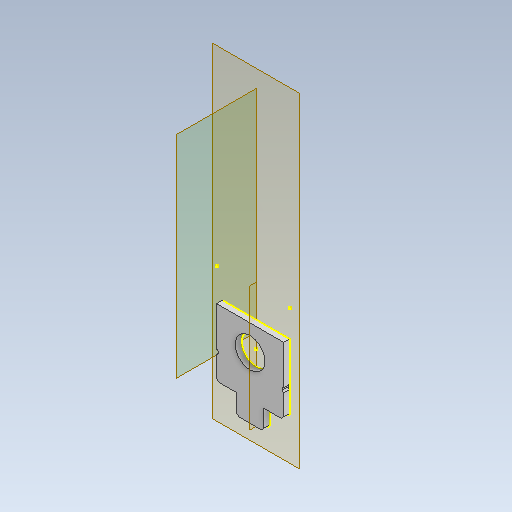
# Autodesk Inventor part: internal
Saved by Autodesk Inventor 2020 (Build 240168000, 168)
## iProperties
Created: 2020-02-17
Part Number: internal
Material: Generic
Document SubType Name: Modeling
Designer: erwin
Density: 1 g/cm^3
Appearance: Default
Mass: 213.639 g
Surface Area: 453.068 cm^2
Volume: 213.639 cm^3
Author: erwin
Autodesk Inventor part; units mm, degrees
ref_plane "YZ Plane" through (0, 0, 0) normal (1, 0, 0) x (0, 1, 0)
ref_plane "XZ Plane" through (0, 0, 0) normal (0, 1, 0) x (-1, 0, 0)
ref_plane "XY Plane" through (0, 0, 0) normal (0, 0, 1) x (1, 0, 0)
ref_plane "Work Plane1" through (0, 0, 0) normal (0, 0, 1) x (1, 0, 0)
sketch "Sketch1" plane through (0, 0, 0) normal (0, 0, 1) x (1, 0, 0)
  circle A0 centre (-67.9848, -106.1458) radius 30 projected
  line L0 (0, -139.7083) -> (0, -24) projected
  line L1 (-95.6323, -230.1458) -> (-40.3675, -230.1458)
  line L2 (-40.3675, -230.1458) -> (-40.3675, -106.1458)
  line L3 (-40.3675, -106.1458) -> (-95.6323, -106.1458)
  line L4 (-95.6323, -106.1458) -> (-95.6323, -230.1458)
  line L5 (-135.9998, -189.7783) -> (0, -189.7783)
  line L6 (0, -189.7783) -> (0, -53.7785)
  line L7 (0, -53.7785) -> (-135.9998, -53.7785)
  line L8 (-135.9998, -53.7785) -> (-135.9998, -189.7783)
  line L9 (-147.9998, -163.7083) -> (-135.9998, -163.7083) projected
  line L10 (-135.9998, -189.7783) -> (-135.9998, -163.7083) projected
  line L11 (-135.9998, -189.7783) -> (-147.9998, -189.7783) projected
  line L12 (-147.9998, -189.7783) -> (-147.9998, -163.7083) projected
  point P0 (0, 0)
  point P1 (-40.3675, -230.1458)
  point P2 (0, -189.7783)
  point P3 (-40.3675, -189.7783)
  point P4 (-95.6323, -189.7783)
  constraints: 16 end point, 4 parallel, 3 perpendicular, 2 collinear, 2 horizontal, 1 point on line, 3 other
extrude "Extrusion1" add sketch "Sketch1" along normal blind 12 contours A0 L4 L5 L8 L7 L0 L6 L2 | A0 L2 L5 L4 | L5 L2 L1 L4
chamfer "Chamfer1" distance 5 angle 45 4 edges at (-135.9998, -189.7783, 6) (-95.6323, -230.1458, 6) (-40.3675, -230.1458, 6) (0, -189.7783, 6)
sketch "Sketch4" plane through (0, 0, 0) normal (0, 0, -1) x (-1, 0, 0)
  line L0 (135.9998, -163.7083) -> (135.9998, -139.7083) projected
  line L1 (135.9998, -136.7194) -> (135.9998, 252.4278) projected
  line L2 (135.9998, -136.7194) -> (135.9998, -139.7083) construction
  line L3 (135.9998, -53.7785) -> (135.9998, -184.7783) projected
  line L4 (132.9998, -136.7194) -> (132.9998, -139.7083)
  line L5 (138.9998, -139.7083) -> (138.9998, -136.7194)
  arc A0 (138.9998, -136.7194) -> (132.9998, -136.7194) centre (135.9998, -136.7194) ccw
  arc A1 (132.9998, -139.7083) -> (138.9998, -139.7083) centre (135.9998, -139.7083) ccw
  point P0 (0, 0)
  point P1 (135.9998, -138.2139)
  point P2 (135.9998, -142.7083)
  point P3 (135.9998, -133.7194)
  dimension "d6" = 6
  constraints: 8 end point, 4 point on circle, 4 tangent, 2 centre point, 1 collinear, 1 midpoint, 1 parallel
  measures "d6" diameter of A1
extrude "Extrusion2" cut sketch "Sketch4" against normal through all contours A1 L4 A0 L1 L3 L0
sketch "Sketch5" plane through (0, 0, 0) normal (0, 0, -1) x (-1, 0, 0)
  arc A0 (135.9998, -133.7194) -> (132.9998, -136.7194) centre (135.9998, -136.7194) ccw projected
  line L0 (135.9998, -53.7785) -> (135.9998, -133.7194) projected
  line L1 (0, -53.7785) -> (135.9998, -53.7785) projected
  line L2 (0, -184.7783) -> (0, -53.7785) projected
  line L3 (5, -189.7783) -> (0, -184.7783) projected
  line L4 (40.3675, -189.7783) -> (5, -189.7783) projected
  line L5 (40.3675, -225.1458) -> (40.3675, -189.7783) projected
  line L6 (45.3675, -230.1458) -> (40.3675, -225.1458) projected
  line L7 (90.6323, -230.1458) -> (45.3675, -230.1458) projected
  line L8 (95.6323, -225.1458) -> (90.6323, -230.1458) projected
  line L9 (95.6323, -189.7783) -> (95.6323, -225.1458) projected
  line L10 (130.9998, -189.7783) -> (95.6323, -189.7783) projected
  line L11 (135.9998, -184.7783) -> (130.9998, -189.7783) projected
  line L12 (135.9998, -142.7083) -> (135.9998, -184.7783) projected
  arc A1 (132.9998, -139.7083) -> (135.9998, -142.7083) centre (135.9998, -139.7083) ccw projected
  line L13 (132.9998, -139.7083) -> (132.9998, -136.7194) projected
  circle A2 centre (67.9848, -106.1458) radius 30 projected
  point P0 (0, 0)
ref_plane "Work Plane2" through (-147.9998, 57.8542, 0) normal (-1, 0, 0) x (0, -1, 0)
sketch "Sketch6" plane through (-147.9998, 57.8542, 0) normal (-1, 0, 0) x (0, -1, 0)
  point P0 (57.8542, 0)
ref_plane "Work Plane3" through (-67.9999, -53.7785, 12) normal (1, 0, 0) x (0, 0, -1)
mirror "Mirror1" about plane through (-67.9999, -53.7785, 12) normal (1, 0, 0) of "Extrusion2"
body "Solid1"
